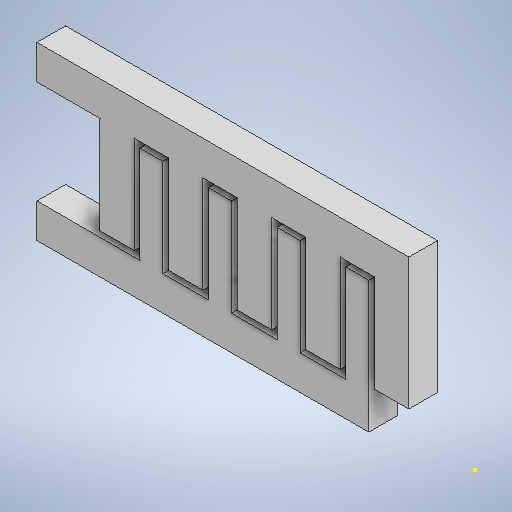
# Autodesk Inventor part: Sensor
Saved by Autodesk Inventor 2025.2 (Build 292293000, 293)
## iProperties
Created: 2025-03-19
Part Number: Sensor
Material: Generic
Document SubType Name: Modeling
Designer: ishad
Density: 1 g/cm^3
Appearance: Default
Author: ishad
Autodesk Inventor part; units mm, degrees
ref_plane "YZ Plane" through (0, 0, 0) normal (1, 0, 0) x (0, 1, 0)
ref_plane "XZ Plane" through (0, 0, 0) normal (0, 1, 0) x (-1, 0, 0)
ref_plane "XY Plane" through (0, 0, 0) normal (0, 0, 1) x (1, 0, 0)
sketch "Sketch1" plane through (0, 0, 0) normal (0, 0, 1) x (1, 0, 0)
  line L0 (-6.5647, 31.3909) -> (-6.5647, 8.3909)
  line L1 (-6.5647, 8.3909) -> (-12.5647, 8.3909)
  line L2 (-18.5647, 8.3909) -> (-24.5647, 8.3909)
  line L3 (-30.5647, 8.3909) -> (-36.5647, 8.3909)
  line L4 (-54.5647, 8.3909) -> (-60.5647, 8.3909)
  line L5 (-6.5647, 31.3909) -> (-71.5647, 31.3909)
  line L6 (-71.5647, 31.3909) -> (-71.5647, 25.3909)
  line L7 (-71.5647, 25.3909) -> (-60.5647, 25.3909)
  line L8 (-60.5647, 25.3909) -> (-60.5647, 8.3909)
  line L9 (-54.5647, 8.3909) -> (-54.5647, 25.3909)
  line L10 (-54.5647, 25.3909) -> (-48.5647, 25.3909)
  line L11 (-48.5647, 25.3909) -> (-48.5647, 8.3909)
  line L12 (-48.5647, 8.3909) -> (-42.5647, 8.3909)
  line L13 (-42.5647, 8.3909) -> (-42.5647, 25.3909)
  line L14 (-42.5647, 25.3909) -> (-36.5647, 25.3909)
  line L15 (-36.5647, 25.3909) -> (-36.5647, 8.3909)
  line L16 (-30.5647, 8.3909) -> (-30.5647, 25.3909)
  line L17 (-30.5647, 25.3909) -> (-24.5647, 25.3909)
  line L18 (-24.5647, 25.3909) -> (-24.5647, 8.3909)
  line L19 (-18.5647, 8.3909) -> (-18.5647, 25.3909)
  line L20 (-18.5647, 25.3909) -> (-12.5647, 25.3909)
  line L21 (-12.5647, 25.3909) -> (-12.5647, 8.3909)
  line L22 (-71.5647, 7.3909) -> (-57.5647, 7.3909)
  line L23 (-71.5647, 7.3909) -> (-71.5647, 1.3909)
  line L24 (-71.5647, 1.3909) -> (-53.5647, 1.3909)
  line L25 (-57.5647, 7.3909) -> (-53.5647, 7.3909)
  line L26 (-53.5647, 7.3909) -> (-53.5647, 24.3909)
  line L27 (-53.5647, 24.3909) -> (-49.5647, 24.3909)
  line L28 (-49.5647, 24.3909) -> (-49.5647, 16.8909)
  line L29 (-49.5647, 16.8909) -> (-49.5647, 7.3909)
  line L30 (-49.5647, 7.3909) -> (-41.5647, 7.3909)
  line L31 (-41.5647, 7.3909) -> (-41.5647, 16.8909)
  line L32 (-41.5647, 24.3909) -> (-41.5647, 16.8909)
  line L33 (-41.5647, 24.3909) -> (-37.5647, 24.3909)
  line L34 (-37.5647, 24.3909) -> (-37.5647, 7.3909)
  line L35 (-53.5647, 1.3909) -> (-13.5647, 1.3909)
  line L36 (-13.5647, 1.3909) -> (-13.5647, 16.8909)
  line L37 (-13.5647, 16.8909) -> (-13.5647, 24.3909)
  line L38 (-13.5647, 24.3909) -> (-17.5647, 24.3909)
  line L39 (-17.5647, 24.3909) -> (-17.5647, 7.3909)
  line L40 (-17.5647, 7.3909) -> (-25.5647, 7.3909)
  line L41 (-25.5647, 7.3909) -> (-25.5647, 24.3909)
  line L42 (-25.5647, 24.3909) -> (-29.5647, 24.3909)
  line L43 (-29.5647, 24.3909) -> (-29.5647, 7.3909)
  line L44 (-29.5647, 7.3909) -> (-37.5647, 7.3909)
  point P0 (0, 0)
  point P1 (-34.0647, 31.3909)
  dimension "d90" = 6
  dimension "d91" = 6
  constraints: 90 end point, 21 perpendicular, 11 horizontal, 9 vertical, 8 point on line, 1 collinear, 1 horizontal alignment
  measures "d90" distance of L22.start L23.end
  measures "d91" distance of L5.end L6.end
sketch "Sketch2" plane through (0, 0, 0) normal (0, 0, 1) x (1, 0, 0)
  point P0 (0, 0)
extrude "Extrusion1" add sketch "Sketch1" along normal blind 5
body "Solid1"
